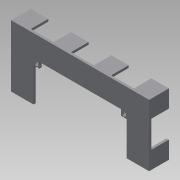
# Autodesk Inventor part: cover back i2c
Saved by Autodesk Inventor 2015 SP1 (Build 190203100, 203)
## iProperties
Created: 2015-04-14
Part Number: cover back i2c
Material: Generic
Document SubType Name: Modeling
Designer: Rafi Kurnia Putra
Density: 1 g/cm^3
Appearance: Default
Author: Rafi Kurnia Putra
Autodesk Inventor part; units mm, degrees
ref_plane "YZ Plane" through (0, 0, 0) normal (1, 0, 0) x (0, 1, 0)
ref_plane "XZ Plane" through (0, 0, 0) normal (0, 1, 0) x (-1, 0, 0)
ref_plane "XY Plane" through (0, 0, 0) normal (0, 0, 1) x (1, 0, 0)
sketch "Sketch1" plane through (0, 0, 0) normal (0, 1, 0) x (-1, 0, 0)
  circle A0 centre (37.593, 4.5441) radius 1.75
  circle A1 centre (-37.593, 4.5441) radius 1.75
  line L0 (-35.093, 7.0441) -> (-35.093, 2.0441)
  circle A2 centre (-37.593, 4.5441) radius 1.75
  line L1 (-35.093, 7.0441) -> (35.093, 7.0441)
  line L2 (35.093, 7.0441) -> (35.093, 2.0441)
  circle A3 centre (37.593, 4.5441) radius 1.75
  line L3 (40.093, 2.0441) -> (40.093, -27.1071)
  line L4 (-40.093, -27.1071) -> (-40.093, 2.0441)
  line L5 (35.093, 2.0441) -> (40.093, 2.0441)
  line L6 (-35.093, 2.0441) -> (-40.093, 2.0441)
  line L7 (-59.2989, -27.1071) -> (-59.2989, 26)
  line L8 (-59.2989, 26) -> (59.2989, 26)
  line L9 (59.2989, 26) -> (59.2989, -27.1071)
  line L10 (59.2989, -27.1071) -> (40.093, -27.1071)
  line L11 (-40.093, -27.1071) -> (-59.2989, -27.1071)
  point P0 (0, 0)
  point P1 (0, 0)
  constraints: 24 end point, 4 centre point, 1 collinear, 1 horizontal, 8 other
extrude "Extrusion1" add sketch "Sketch1" along normal blind 3
sketch "Sketch3" plane through (0, 3, 0) normal (0, 1, 0) x (1, 0, 0)
  line L0 (-59.2989, -26) -> (-59.2989, -11)
  line L1 (-59.2989, 27.1071) -> (-59.2989, -26) projected
  line L2 (-59.2989, -26) -> (-44.2989, -26)
  line L3 (-59.2989, -26) -> (59.2989, -26) projected
  line L4 (-59.2989, -11) -> (-57.2989, -11)
  line L5 (-57.2989, -11) -> (-57.2989, -24)
  line L6 (-57.2989, -24) -> (-44.2989, -24)
  line L7 (-44.2989, -24) -> (-44.2989, -26)
  line L8 (0, 0) -> (0, 7) construction
  line L9 (59.2989, -26) -> (59.2989, -11)
  line L10 (59.2989, -26) -> (44.2989, -26)
  line L11 (59.2989, -11) -> (57.2989, -11)
  line L12 (57.2989, -11) -> (57.2989, -24)
  line L13 (57.2989, -24) -> (44.2989, -24)
  line L14 (44.2989, -24) -> (44.2989, -26)
  line L15 (-24.7663, -26) -> (-24.7663, -24)
  line L16 (-24.7663, -24) -> (-9.7663, -24)
  line L17 (-9.7663, -24) -> (-9.7663, -26)
  line L18 (-24.7663, -26) -> (-9.7663, -26)
  line L19 (24.7663, -26) -> (9.7663, -26)
  line L20 (9.7663, -26) -> (9.7663, -24)
  line L21 (9.7663, -24) -> (24.7663, -24)
  line L22 (24.7663, -24) -> (24.7663, -26)
  line L23 (-59.2989, 27.1071) -> (-59.2989, 12.1071)
  line L24 (-59.2989, 12.1071) -> (-57.2989, 12.1071)
  line L25 (-57.2989, 12.1071) -> (-57.2989, 27.1071)
  line L26 (-40.093, 27.1071) -> (-59.2989, 27.1071) projected
  line L27 (-59.2989, 27.1071) -> (-57.2989, 27.1071)
  line L28 (59.2989, 27.1071) -> (59.2989, 12.1071)
  line L29 (59.2989, 12.1071) -> (57.2989, 12.1071)
  line L30 (57.2989, 12.1071) -> (57.2989, 27.1071)
  line L31 (59.2989, 27.1071) -> (57.2989, 27.1071)
  dimension "d3" = 15
  dimension "d4" = 2
  dimension "d5" = 88.5979
  dimension "d6" = 19.5327
  dimension "d7" = 15
  dimension "d8" = 19.5327
  dimension "d9" = 15
  dimension "d10" = 2
  dimension "d11" = 15
  dimension "d12" = 2
  dimension "d15" = 2
  dimension "d16" = 2
  constraints: 58 end point, 11 perpendicular, 9 symmetric about line, 8 point on line, 2 collinear, 2 vertical
  measures "d3" distance of L0.start L2.end
  measures "d4" distance of L0.end L4.end
  measures "d5" distance between parallel lines of L14 L7
  measures "d6" distance of L15.start L2.end
  measures "d7" distance of L15.end L16.end
  measures "d8" distance of L19.start L10.end
  measures "d9" distance of L19.start L19.end
  measures "d10" distance of L19.end L20.end
  measures "d11" distance of L1.start L23.end
  measures "d12" distance of L23.end L24.end
  measures "d15" distance between parallel lines of L3 L6
  measures "d16" distance between parallel lines of L3 L16
extrude "Extrusion2" add sketch "Sketch3" along normal blind 15
sketch "Sketch5" plane through (0, 0, 0) normal (0, -1, 0) x (1, 0, 0)
  circle A0 centre (37.593, 4.5441) radius 1.75 projected
  circle A1 centre (-37.593, 4.5441) radius 1.75 projected
  line L0 (-59.2989, -27.1071) -> (-40.093, -27.1071) projected
  line L1 (-40.093, -27.1071) -> (-40.093, 2.0441) projected
  line L2 (-40.093, 2.0441) -> (-35.093, 2.0441) projected
  line L3 (-35.093, 2.0441) -> (-35.093, 7.0441) projected
  line L4 (-35.093, 7.0441) -> (35.093, 7.0441) projected
  line L5 (35.093, 7.0441) -> (35.093, 2.0441) projected
  line L6 (35.093, 2.0441) -> (40.093, 2.0441) projected
  line L7 (40.093, 2.0441) -> (40.093, -27.1071) projected
  line L8 (40.093, -27.1071) -> (59.2989, -27.1071) projected
  line L9 (59.2989, -27.1071) -> (59.2989, 26) projected
  line L10 (59.2989, 26) -> (-59.2989, 26) projected
  line L11 (-59.2989, 26) -> (-59.2989, -27.1071) projected
  point P0 (0, 0)
extrude "Extrusion3" cut sketch "Sketch5" against normal blind 1
body "Solid1"
